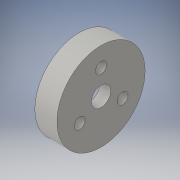
# Autodesk Inventor part: Figure 6_16_N
Saved by Autodesk Inventor 2016 (Build 200138000, 138)
## iProperties
Created: 2016-07-21
Part Number: Figure 6_16_N
Material: Generic
Document SubType Name: Modeling
Designer: cfkguest
Density: 1 g/cm^3
Appearance: Default
Author: cfkguest
Autodesk Inventor part; units mm, degrees
ref_plane "YZ Plane" through (0, 0, 0) normal (1, 0, 0) x (0, 1, 0)
ref_plane "XZ Plane" through (0, 0, 0) normal (0, 1, 0) x (-1, 0, 0)
ref_plane "XY Plane" through (0, 0, 0) normal (0, 0, 1) x (1, 0, 0)
sketch "Sketch1" plane through (0, 0, 0) normal (0, 1, 0) x (-1, 0, 0)
  line L0 (0, 0) -> (-101.6, 0)
  line L1 (-84.1264, -11.176) -> (-84.1264, -50.8)
  line L2 (-84.1264, -50.8) -> (-58.7264, -50.8)
  line L3 (-58.7264, -50.8) -> (-58.7264, -44.45)
  line L4 (-58.7264, -44.45) -> (-71.4264, -44.45)
  line L5 (-71.4264, -44.45) -> (-71.4264, -11.176)
  line L6 (-71.4264, -11.176) -> (-84.1264, -11.176)
  dimension "d0" = 101.6
  dimension "d1" = 11.176
  dimension "d2" = 50.8
  dimension "d3" = 6.35
  dimension "d4" = 25.4
  dimension "d5" = 12.7
  dimension "d6" = 71.4264
  constraints: 14 end point, 5 perpendicular, 1 horizontal, 1 vertical
  measures "d0" distance of L0.start L0.end
  measures "d1" distance between parallel lines of L0 L6
  measures "d2" distance between parallel lines of L0 L2
  measures "d3" distance of L2.end L3.end
  measures "d4" distance of L1.end L2.end
  measures "d5" distance of L3.end L4.end
  measures "d6" horizontal distance of L0.start L5.end
revolve "Revolution1" add sketch "Sketch1" angle 360 about axis through (0, 0, 0) along (1, 0, 0)
sketch "Sketch2" plane through (71.4264, 0, 0) normal (-1, 0, 0) x (0, 0, 1)
  circle A0 centre (0, 0) radius 28.575
  point P0 (0, 28.575)
  point P1 (-24.7467, -14.2875)
  point P2 (24.7467, -14.2875)
  dimension "d8" = 57.15
  dimension "d11" = 360
  constraints: 1 coincident, 1 vertical alignment, 6 other
hole "Hole1" at (71.4264, 28.575, 0) at (71.4264, -14.2875, -24.7467) at (71.4264, -14.2875, 24.7467) direction (1, 0, 0) diameter 12.7 end through all
body "Solid1"
